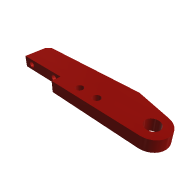
# Autodesk Inventor part: 100016
Saved by Autodesk Inventor 2020.1 (Build 241239000, 239)
## iProperties
Company: AUTODESK, INC.
Part Number: 100016
Document SubType Name: Modeling
Created: 2004-04-01
Designer: SCHNEIDER K.
Material: STEEL - HIGH GRADE ALLOY
Project: ADSK-000-000000
Description: ARM
Density: 7.86 g/cm^3
Appearance: Orange-Red
Control State: 0
Master: False
Checked Out: False
Shininess: 64.0
Length Units: 11269
Angle Units: 11279
Time Units: 11290
Mass Units: 11283
Length Display Precision: 3
Angle Display Precision: 2
Compacted: True
Density: 0.0
Volumn: 0.0
Area: 0.0
PropertySet Name: Model Information
Title: PLATE
Author: SCHNEIDER K.
Revision Number: -
Autodesk Inventor part; units mm, degrees
ref_plane "YZ Plane" through (0, 0, 0) normal (1, 0, 0) x (0, 1, 0)
ref_plane "XZ Plane" through (0, 0, 0) normal (0, 1, 0) x (-1, 0, 0)
sketch "スケッチ2" plane through (0, 0, 0) normal (0, 0, 1) x (1, 0, 0)
  line L0 (-13.5609, 243.4507) -> (-13.5609, 273.4507)
  line L1 (-13.5609, 273.4507) -> (136.4391, 273.4507)
  arc A0 (136.4391, 243.4507) -> (136.4391, 273.4507) centre (136.4391, 258.4507) ccw
  line L2 (136.4391, 243.4507) -> (-13.5609, 243.4507)
  point P0 (0, 0)
  dimension "d15" = 15
  dimension "d48" = 150
  constraints: 6 end point, 2 point on circle, 2 point on line, 2 tangent, 1 centre point, 1 parallel, 1 perpendicular, 1 vertical
  measures "d15" radius of A0
  measures "d48" distance from line of L0 A0.centre
extrude "押し出し2" add sketch "スケッチ2" against normal blind 12
sketch "スケッチ3" plane through (0, 0, 0) normal (0, 0, 1) x (1, 0, 0)
  arc A0 (136.4391, 273.4507) -> (136.4391, 243.4507) centre (136.4391, 258.4507) ccw projected
  point P0 (86.4391, 253.4507)
  point P1 (66.4391, 253.4507)
  dimension "d4" = 20
  dimension "d5" = 50
  dimension "d6" = 5
  constraints: 1 horizontal alignment
  measures "d4" distance of point (66.439, 253.451) point (86.439, 253.451)
  measures "d5" horizontal distance of A0.centre point (86.439, 253.451)
  measures "d6" vertical distance of A0.centre point (86.439, 253.451)
hole "穴1" at (86.4391, 253.4507, 0) at (66.4391, 253.4507, 0) direction (0, 0, -1) diameter 8 end through all
sketch "スケッチ4" plane through (0, 0, -12) normal (0, 0, -1) x (-1, 0, 0)
  arc A0 (-136.4391, 273.4507) -> (-136.4391, 243.4507) centre (-136.4391, 258.4507) ccw projected
  constraints: 1 coincident
hole "穴2" at (136.4391, 258.4507, -12) direction (0, 0, 1) diameter 14 end through all
sketch "スケッチ7" plane through (0, 0, 0) normal (0, 0, 1) x (1, 0, 0)
  arc A0 (136.4391, 243.4507) -> (136.4391, 273.4507) centre (136.4391, 258.4507) ccw projected
  line L0 (136.4391, 273.4507) -> (-13.5609, 273.4507) projected
  line L1 (-13.5609, 243.4507) -> (136.4391, 243.4507) projected
  line L2 (-13.5609, 273.4507) -> (-13.5609, 283.4507)
  line L3 (-13.5609, 283.4507) -> (106.4391, 283.4507)
  line L4 (106.4391, 283.4507) -> (140.879, 272.7786)
  dimension "d49" = 10
  dimension "d50" = 120
  constraints: 6 end point, 2 perpendicular, 1 point on circle, 1 tangent
  measures "d49" distance of L0.end L2.end
  measures "d50" distance of L2.end L3.end
extrude "押し出し3" add sketch "スケッチ7" against normal up to surface (12 mm away)
sketch "スケッチ8" plane through (0, 0, 0) normal (0, 0, 1) x (1, 0, 0)
  line L0 (-13.5609, 243.4507) -> (41.4391, 243.4507)
  line L1 (41.4391, 243.4507) -> (41.4391, 253.4507)
  line L2 (41.4391, 253.4507) -> (-13.5609, 253.4507)
  line L3 (-13.5609, 253.4507) -> (-13.5609, 243.4507)
  dimension "d53" = 10
  dimension "d54" = 55
  constraints: 8 end point, 2 parallel, 1 horizontal, 1 perpendicular
  measures "d53" distance of L2.end L0.start
  measures "d54" distance of L1.end L2.end
extrude "押し出し4" cut sketch "スケッチ8" against normal through all
sketch "スケッチ9" plane through (-13.5609, 253.4507, 0) normal (0, -1, 0) x (1, 0, 0)
  line L0 (55, 0) -> (55, -12) projected
  line L1 (0, -12) -> (0, 0) projected
  line L2 (0, -6) -> (55, -6)
  point P0 (10, -6)
  point P1 (45, -6)
  dimension "d57" = 10
  dimension "d58" = 35
  constraints: 2 end point, 2 midpoint, 1 horizontal alignment, 1 point on line
  measures "d57" distance from line of point (10, -6) L1
  measures "d58" distance of point (45, -6) point (10, -6)
hole "穴5" at (-3.5609, 253.4507, -6) at (31.4391, 253.4507, -6) direction (0, 1, 0) diameter 6.6 end through all
chamfer "面取り1" distance 5 angle 45 1 edges at (-13.5609, 283.4507, -6)
ref_plane "Work Plane1" through (0, 0, -6) normal (0, 0, -1) x (-1, 0, 0)
body "Solid1"
